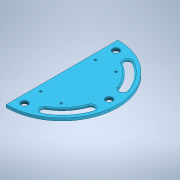
# Autodesk Inventor part: Base 2
Saved by Autodesk Inventor 2020 (Build 240168000, 168)
## iProperties
Created: 2020-10-28
Part Number: Base 2
Material: PC/ABS Plastic
Document SubType Name: Modeling
Designer: aaron
Density: 0.357273 g/cm^3
Appearance: Turquoise
Author: aaron
## iProperties of the stored document _3DPrint.ipt
Created: 2020-11-03
Part Number: _3DPrint
Material: Generic
Document SubType Name: Modeling
Designer: aaron
Density: 1 g/cm^3
Appearance: Default
Author: aaron
Autodesk Inventor part; units mm, degrees
ref_plane "YZ Plane" through (0, 0, 0) normal (1, 0, 0) x (0, 1, 0)
ref_plane "XZ Plane" through (0, 0, 0) normal (0, 1, 0) x (-1, 0, 0)
ref_plane "XY Plane" through (0, 0, 0) normal (0, 0, 1) x (1, 0, 0)
sketch "Sketch1" plane through (0, 0, 0) normal (0, 1, 0) x (-1, 0, 0)
  circle A0 centre (0, 0) radius 41.5 construction
  line L0 (0, -41.5) -> (0, 41.5)
  arc A1 (0, 41.5) -> (0, -41.5) centre (0, 0) ccw
  circle A2 centre (-6, -34) radius 2.5
  circle A3 centre (-6, 34) radius 2.5
  line L1 (0, 0) -> (-41.5, 0) construction
  circle A4 centre (-35, 0) radius 2.5
  circle A5 centre (0, 0) radius 35.5 construction
  line L2 (0, 0) -> (-20.75, -35.9401) construction
  line L3 (0, 0) -> (-38.9972, -14.1938) construction
  arc A6 (-33.3591, -12.1417) -> (-17.75, -30.7439) centre (0, 0) ccw construction
  arc A7 (-35.7083, -12.9968) -> (-19, -32.909) centre (0, 0) ccw
  arc A8 (-31.0099, -11.2867) -> (-16.5, -28.5788) centre (0, 0) ccw
  arc A9 (-31.0099, -11.2867) -> (-35.7083, -12.9968) centre (-33.3591, -12.1417) ccw
  arc A10 (-19, -32.909) -> (-16.5, -28.5788) centre (-17.75, -30.7439) ccw
  arc A11 (-19, 32.909) -> (-35.7083, 12.9968) centre (0, 0) ccw
  arc A12 (-16.5, 28.5788) -> (-31.0099, 11.2867) centre (0, 0) ccw
  arc A13 (-35.7083, 12.9968) -> (-31.0099, 11.2867) centre (-33.3591, 12.1417) ccw
  arc A14 (-16.5, 28.5788) -> (-19, 32.909) centre (-17.75, 30.7439) ccw
  dimension "d2" = 83
  dimension "d3" = 83
  dimension "d4" = 5
  dimension "d5" = 6
  dimension "d6" = 34
  dimension "d7" = 34
  dimension "d8" = 35
  dimension "d11" = 6
  dimension "d12" = 20
  dimension "d13" = 30
  dimension "d14" = 5
  constraints: 27 point on circle, 15 centre point, 8 end point, 6 symmetric about line, 4 equal radius, 4 tangent, 3 coincident, 3 point on line, 1 midpoint, 1 vertical, 1 vertical alignment, 4 other
  measures "d2" diameter of A0
  measures "d3" distance of L0.start L0.end
  measures "d4" diameter of A2
  measures "d5" horizontal distance of point (0, 0) A2.centre
  measures "d6" vertical distance of point (0, 0) A2.centre
  measures "d7" vertical distance of point (0, 0) A3.centre
  measures "d8" distance of point (0, 0) A4.centre
  measures "d11" radial gap between concentric circles of A0 A5
  measures "d12" angle of L1 L3
  measures "d13" angle of L2 L0
  measures "d14" diameter of A9
extrude "Extrusion1" add sketch "Sketch1" along normal blind 2
sketch "Dimen. Arduino" plane through (0, 2, 0) normal (0, 1, 0) x (1, 0, 0)
  line L0 (0, 0) -> (41.5, 0) construction
  arc A0 (0, -41.5) -> (0, 41.5) centre (0, 0) ccw construction
  line L1 (3.11, -21.59) -> (20.89, -21.59) construction
  line L2 (20.89, -21.59) -> (20.89, 21.59) construction
  line L3 (20.89, 21.59) -> (3.11, 21.59) construction
  line L4 (3.11, 21.59) -> (3.11, -21.59) construction
  line L5 (3.11, -21.59) -> (20.89, 21.59) construction
  line L6 (20.89, -21.59) -> (3.11, 21.59) construction
  line L7 (19.62, -20.32) -> (4.38, -20.32) construction
  line L8 (4.38, -20.32) -> (4.38, 20.32) construction
  line L9 (4.38, 20.32) -> (19.62, 20.32) construction
  line L10 (19.62, 20.32) -> (19.62, -20.32) construction
  line L11 (19.62, -20.32) -> (4.38, 20.32) construction
  line L12 (4.38, -20.32) -> (19.62, 20.32) construction
  circle A1 centre (4.38, 20.32) radius 0.75
  circle A2 centre (19.62, 20.32) radius 0.75
  circle A3 centre (4.38, -20.32) radius 0.75
  circle A4 centre (19.62, -20.32) radius 0.75
  point P0 (12, 0)
  dimension "d17" = 43.18
  dimension "d18" = 17.78
  dimension "d19" = 12
  dimension "d20" = 1.27
  dimension "d21" = 1.27
  dimension "d22" = 1.5
  constraints: 26 end point, 4 centre point, 4 coincident, 4 midpoint, 4 parallel, 3 equal radius, 3 horizontal, 2 perpendicular, 1 point on circle, 1 point on line
  measures "d17" distance of L3.end L1.start
  measures "d18" distance of L2.end L3.end
  measures "d19" distance of point (12, 0) L0.start
  measures "d20" distance between parallel lines of L9 L3
  measures "d21" distance between parallel lines of L2 L10
  measures "d22" diameter of A1
extrude "Extrusion2" cut sketch "Dimen. Arduino" against normal through all
fillet "Fillet1" radius 1 16 edges at (25.2795, 2, 21.212) (34.2141, 2, 9.7925) (29.1097, 2, 24.4259) (15.5849, 2, 31.9939) (15.5849, 2, -31.9939) (29.1097, 2, -24.4259) (34.2141, 2, -9.7925) (25.2795, 2, -21.212) (29.1097, 0, 24.4259) (15.5849, 0, 31.9939) (25.2795, 0, 21.212) (34.2141, 0, 9.7925) (25.2795, 0, -21.212) (15.5849, 0, -31.9939) (29.1097, 0, -24.4259) (34.2141, 0, -9.7925)
body "Solid1"
